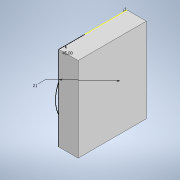
# Autodesk Inventor part: battery holder
Saved by Autodesk Inventor 2020 (Build 240168000, 168)
## iProperties
Created: 2020-07-25
Part Number: battery holder
Material: Generic
Document SubType Name: Modeling
Designer: franc
Density: 1 g/cm^3
Appearance: Default
Author: franc
Autodesk Inventor part; units mm, degrees
ref_plane "YZ Plane" through (0, 0, 0) normal (1, 0, 0) x (0, 1, 0)
ref_plane "XZ Plane" through (0, 0, 0) normal (0, 1, 0) x (-1, 0, 0)
ref_plane "XY Plane" through (0, 0, 0) normal (0, 0, 1) x (1, 0, 0)
sketch "Sketch1" plane through (0, 0, 0) normal (0, 0, 1) x (1, 0, 0)
  line L0 (-3, -13) -> (3, -13)
  line L1 (3, -13) -> (3, 13)
  line L2 (3, 13) -> (-3, 13)
  line L3 (-3, 13) -> (-3, -13)
  line L4 (-3, -13) -> (3, 13) construction
  line L5 (3, -13) -> (-3, 13) construction
  line L6 (0, 13) -> (0, -13) construction
  circle A0 centre (0, 8.25) radius 1.25
  circle A1 centre (0, -8.25) radius 1.25
  line L7 (-4.2, 0) -> (4.2, 0) construction
  circle A2 centre (0, 8.25) radius 3 construction
  circle A3 centre (0, -8.25) radius 3 construction
  line L8 (-0.775, -0.425) -> (0.775, -0.425) construction
  line L9 (0.775, -0.425) -> (0.775, 0.425) construction
  line L10 (0.775, 0.425) -> (-0.775, 0.425) construction
  line L11 (-0.775, 0.425) -> (-0.775, -0.425) construction
  line L12 (-0.775, -0.425) -> (0.775, 0.425) construction
  line L13 (0.775, -0.425) -> (-0.775, 0.425) construction
  line L14 (-0.9, -0.55) -> (0.9, -0.55)
  line L15 (0.9, -0.55) -> (0.9, 0.55)
  line L16 (0.9, 0.55) -> (-0.9, 0.55)
  line L17 (-0.9, 0.55) -> (-0.9, -0.55)
  line L18 (-0.9, -0.55) -> (0.9, 0.55) construction
  line L19 (0.9, -0.55) -> (-0.9, 0.55) construction
  point P0 (0, 0)
  dimension "d0" = 2.5
  dimension "d1" = 2.5
  dimension "d2" = 16.5
  dimension "d3" = 26
  dimension "d4" = 6
  dimension "d5" = 0.85
  dimension "d6" = 1.55
  dimension "d7" = 1.8
  dimension "d8" = 1.1
  constraints: 38 end point, 8 midpoint, 6 parallel, 4 centre point, 3 horizontal, 3 perpendicular, 2 coincident, 2 point on line, 2 tangent, 1 symmetric about line
  measures "d0" diameter of A0
  measures "d1" diameter of A1
  measures "d2" distance of A1.centre A0.centre
  measures "d3" distance between parallel lines of L0 L2
  measures "d4" distance between parallel lines of L3 L1
  measures "d5" distance of L8.end L9.end
  measures "d6" distance of L9.end L10.end
  measures "d7" distance of L16.end L15.end
  measures "d8" distance of L14.end L15.end
extrude "Extrusion1" add sketch "Sketch1" along normal blind 21
sketch "Sketch7" plane through (0, 0, 21) normal (0, 0, 1) x (1, 0, 0)
  line L0 (3, 13) -> (-3, 13) projected
  line L1 (-3, 13) -> (3, 13)
  line L2 (3, 13) -> (3, -13)
  line L3 (3, -13) -> (-3, -13)
  line L4 (-3, -13) -> (-3, 13)
  point P0 (0, 0)
  constraints: 8 end point, 2 parallel, 1 coincident, 1 horizontal, 1 perpendicular
extrude "Extrusion4" add sketch "Sketch7" against normal blind 15
sketch "Sketch6" plane through (-3, -13, 0) normal (-1, 0, 0) x (0, 0, 1)
  line L0 (0, 13) -> (21.1523, 13) construction
  line L1 (0, 12.45) -> (21, 12.45) construction
  circle A0 centre (11.5, 13) radius 10.5
  line L2 (1, 25.8726) -> (1, 0) construction
  line L3 (0, 0) -> (21, 0) projected
  line L4 (0, 26) -> (0, 0) construction
  line L5 (17.2376, 21.7937) -> (13.0314, 26)
  line L6 (0, 26) -> (21, 26) projected
  line L7 (13.0314, 26) -> (21, 26)
  line L8 (21, 0) -> (21, 26) projected
  line L9 (21, 26) -> (21, 0)
  dimension "d25" = 21
  dimension "d26" = 1
  dimension "d29" = 45
  constraints: 10 end point, 3 point on line, 3 vertical, 1 horizontal, 1 parallel, 3 other
  measures "d26" distance between parallel lines of L4 L2
  measures "d29" angle of L6 L5
sketch "Sketch3" plane through (-3, 13, 0) normal (0, 1, 0) x (1, 0, 0)
  line L0 (6, -4.4) -> (0, -4.4)
  line L1 (0, -4.4) -> (0, -1.9)
  line L2 (0, -1.9) -> (6, -1.9)
  line L3 (6, -1.9) -> (6, -4.4)
  line L4 (6, 0) -> (6, -21) projected
  line L5 (0, 0) -> (0, -21) projected
  line L6 (6, 0) -> (0, 0) projected
  point P0 (3, 0)
  dimension "d14" = 4.4
  dimension "d15" = 2.5
  constraints: 8 end point, 2 collinear, 2 parallel, 1 horizontal, 1 perpendicular
  measures "d14" distance between parallel lines of L6 L0
  measures "d15" distance between parallel lines of L0 L2
sketch "Sketch4" plane through (-3, 13, 1.9) normal (0, 0, 1) x (1, 0, 0)
  circle A0 centre (3, -4.75) radius 1.5 projected
  line L0 (1.4123, -2) -> (4.5877, -2)
  line L1 (4.5877, -2) -> (6.1754, -4.75)
  line L2 (6.1754, -4.75) -> (4.5877, -7.5)
  line L3 (4.5877, -7.5) -> (1.4123, -7.5)
  line L4 (1.4123, -7.5) -> (-0.1754, -4.75)
  line L5 (-0.1754, -4.75) -> (1.4123, -2)
  line L6 (6, 0) -> (0, 0) projected
  line L7 (3.9, -12.45) -> (3.9, -13.55) projected
  line L8 (3.9, -13.55) -> (2.1, -13.55) projected
  line L9 (3.9, -12.45) -> (2.1, -13.55) construction
  line L10 (0, 0) -> (0, -26) projected
  line L11 (6, -18.4) -> (0, -18.4)
  line L12 (0, -18.4) -> (0, -7.6)
  line L13 (0, -7.6) -> (6, -7.6)
  line L14 (6, -7.6) -> (6, -18.4)
  line L15 (6, -18.4) -> (0, -7.6) construction
  line L16 (0, -18.4) -> (6, -7.6) construction
  line L17 (2.1, -13.55) -> (3.9, -13.55)
  line L18 (3.9, -13.55) -> (3.9, -12.45)
  line L19 (3.9, -12.45) -> (2.1, -12.45)
  line L20 (2.1, -12.45) -> (2.1, -13.55)
  line L21 (2.1, -13.55) -> (3.9, -12.45) construction
  line L22 (3.9, -13.55) -> (2.1, -12.45) construction
  point P0 (3, -13)
  point P1 (0, -18.4)
  dimension "d18" = 5.5
  dimension "d19" = 0.1
  dimension "d23" = 21
  dimension "d12" = 2
  constraints: 4 end point, 2 point on line, 1 horizontal alignment, 1 midpoint, 1 perpendicular, 1 vertical, 2 other
  measures "d12" distance between parallel lines of L4 L2
body "Solid1"
